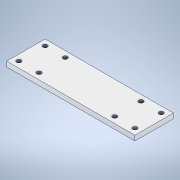
# Autodesk Inventor part: Placa_soporte_chumasera
Saved by Autodesk Inventor 2020 (Build 240168000, 168)
## iProperties
Created: 2021-01-15
Part Number: Placa_soporte_chumasera
Material: Aluminio 6061
Document SubType Name: Modeling
Designer: Cerberus 1S
Density: 2.7 g/cm^3
Appearance: Aluminio - Plano
Author: Cerberus 1S
Autodesk Inventor part; units mm, degrees
ref_plane "YZ Plane" through (0, 0, 0) normal (1, 0, 0) x (0, 1, 0)
ref_plane "XZ Plane" through (0, 0, 0) normal (0, 1, 0) x (-1, 0, 0)
ref_plane "XY Plane" through (0, 0, 0) normal (0, 0, 1) x (1, 0, 0)
sketch "Boceto1" plane through (0, 0, 0) normal (0, 1, 0) x (-1, 0, 0)
  line L0 (0, 0) -> (127, 0)
  line L1 (127, 0) -> (127, -38)
  line L2 (127, -38) -> (0, -38)
  line L3 (0, -38) -> (0, 0)
  dimension "d0" = 127
  dimension "d1" = 38
  constraints: 8 end point, 2 parallel, 1 horizontal, 1 perpendicular
  measures "d0" distance of L1.end L2.end
  measures "d1" distance between parallel lines of L2 L0
extrude "Extrusión1" add sketch "Boceto1" along normal blind 5
sketch "Boceto2" plane through (0, 5, 0) normal (0, 1, 0) x (1, 0, 0)
  line L0 (-127, 38) -> (-127, 0) projected
  line L1 (0, 38) -> (-127, 38) projected
  line L2 (0, 0) -> (0, 38) projected
  line L3 (-127, 0) -> (0, 0) projected
  point P0 (-121, 6)
  point P1 (-101, 6)
  point P2 (-101, 32)
  point P3 (-121, 32)
  point P4 (-26, 6)
  point P5 (-6, 6)
  point P6 (-26, 32)
  point P7 (-6, 32)
  dimension "d4" = 6
  dimension "d5" = 6
  dimension "d6" = 6
  dimension "d7" = 6
  dimension "d8" = 6
  dimension "d9" = 6
  dimension "d10" = 20
  dimension "d11" = 20
  dimension "d12" = 6
  constraints: 4 horizontal alignment, 4 vertical alignment
  measures "d4" distance from line of point (-121, 32) L0
  measures "d5" distance from line of L1 point (-121, 32)
  measures "d6" distance from line of L2 point (-6, 32)
  measures "d7" distance from line of L1 point (-6, 32)
  measures "d8" distance from line of L2 point (-6, 6)
  measures "d9" distance from line of L3 point (-6, 6)
  measures "d10" distance of point (-101, 6) point (-121, 6)
  measures "d11" distance of point (-6, 6) point (-26, 6)
  measures "d12" distance from line of L3 point (-121, 6)
hole "Agujero1" at (-121, 5, -6) at (-101, 5, -6) at (-101, 5, -32) at (-121, 5, -32) at (-26, 5, -6) at (-6, 5, -6) at (-26, 5, -32) at (-6, 5, -32) direction (0, -1, 0) diameter 4.4587 depth 40 tip angle 118 thread size "M5x0.5" class "6H" standard "ANSI Metric M Profile"
